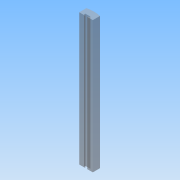
# Autodesk Inventor part: Tunel_IRBeam
Saved by Autodesk Inventor 2016 (Build 200138000, 138)
## iProperties
Created: 2014-11-25
Part Number: Tunel_IRBeam
Material: Acetalharz, schwarz
Document SubType Name: Modeling
Designer: Gero Hofmann
Density: 1.425 g/cm^3
Appearance: Glatt - schwarz
Author: Gero Hofmann
Autodesk Inventor part; units mm, degrees
ref_plane "YZ Plane" through (0, 0, 0) normal (1, 0, 0) x (0, 1, 0)
ref_plane "XZ Plane" through (0, 0, 0) normal (0, 1, 0) x (-1, 0, 0)
ref_plane "XY Plane" through (0, 0, 0) normal (0, 0, 1) x (1, 0, 0)
sketch "Skizze1" plane through (0, 0, 0) normal (0, 0, 1) x (1, 0, 0)
  line L0 (17, 0) -> (17, 18)
  line L1 (-17, 18) -> (-17, 0)
  arc A0 (17, 18) -> (-17, 18) centre (0, -53.25) ccw
  line L2 (-6.5, 4.6) -> (6.5, 4.6)
  line L3 (6.5, 4.6) -> (6.5, 1.6)
  line L4 (-6.5, 1.6) -> (-6.5, 4.6)
  line L5 (-6.5, 4.6) -> (6.5, 1.6) construction
  line L6 (6.5, 4.6) -> (-6.5, 1.6) construction
  line L7 (-3.1, 1.6) -> (-3.1, 0)
  line L8 (3.1, 1.6) -> (3.1, 0)
  line L9 (6.5, 1.6) -> (3.1, 1.6)
  line L10 (-3.1, 1.6) -> (-6.5, 1.6)
  line L11 (-17, 0) -> (-3.1, 0)
  line L12 (3.1, 0) -> (17, 0)
  line L13 (0, 3.1) -> (0, 0) construction
  dimension "d2" = 18
  dimension "d4" = 34
  dimension "d5" = 6.2
  dimension "d6" = 4.6
  dimension "d7" = 3
  dimension "d8" = 13
  dimension "d9" = 20
  constraints: 28 end point, 6 perpendicular, 5 parallel, 4 midpoint, 3 horizontal, 2 collinear, 2 point on circle, 1 centre point, 1 coincident, 1 horizontal alignment, 1 point on line, 2 other
  measures "d2" distance of L1.start L1.end
  measures "d4" distance of L1.end L0.start
  measures "d5" distance between parallel lines of L8 L7
  measures "d6" distance between parallel lines of L12 L2
  measures "d7" distance of L4.start L2.start
  measures "d8" distance of L2.start L2.end
  measures "d9" distance edge to line of A0 L12
extrude "Extrusion1" add sketch "Skizze1" along normal blind 330
